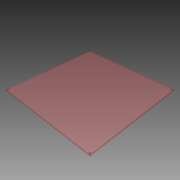
# Autodesk Inventor part: pcb_heatbed
Saved by Autodesk Inventor 2014 (Build 180170000, 170)
## iProperties
Created: 2013-11-29
Part Number: pcb_heatbed
Material: Generic
Document SubType Name: Modeling
Designer: buben
Density: 1 g/cm^3
Appearance: pcb_red
Author: buben
Autodesk Inventor part; units mm, degrees
ref_plane "YZ Plane" through (0, 0, 0) normal (1, 0, 0) x (0, 1, 0)
ref_plane "XZ Plane" through (0, 0, 0) normal (0, 1, 0) x (-1, 0, 0)
ref_plane "XY Plane" through (0, 0, 0) normal (0, 0, 1) x (1, 0, 0)
sketch "Sketch1" plane through (0, 0, 0) normal (0, 0, 1) x (1, 0, 0)
  line L0 (0, 0) -> (214, 0)
  line L1 (214, 0) -> (214, 214)
  line L2 (214, 214) -> (0, 214)
  line L3 (0, 214) -> (0, 0)
  line L4 (2.5, 211.5) -> (211.5, 211.5) construction
  line L5 (211.5, 211.5) -> (211.5, 2.5) construction
  line L6 (211.5, 2.5) -> (2.5, 2.5) construction
  line L7 (2.5, 2.5) -> (2.5, 211.5) construction
  circle A0 centre (2.5, 211.5) radius 1.7
  circle A1 centre (211.5, 211.5) radius 1.7
  circle A2 centre (211.5, 2.5) radius 1.7
  circle A3 centre (2.5, 2.5) radius 1.7
  point P0 (2.5, 107)
  point P1 (0, 107)
  point P2 (107, 211.5)
  point P3 (107, 214)
  dimension "d0" = 214
  dimension "d1" = 214
  dimension "d2" = 3.4
  dimension "d3" = 3.4
  dimension "d4" = 3.4
  dimension "d5" = 3.4
  dimension "d6" = 209
  dimension "d7" = 209
  constraints: 16 end point, 4 centre point, 4 coincident, 4 midpoint, 4 parallel, 2 horizontal, 2 perpendicular, 1 horizontal alignment, 1 vertical alignment
  measures "d0" distance of L0.start L0.end
  measures "d1" distance of L2.end L0.start
  measures "d2" diameter of A3
  measures "d3" diameter of A2
  measures "d4" diameter of A1
  measures "d5" diameter of A0
  measures "d6" distance of L4.start L4.end
  measures "d7" distance of L6.end L4.start
extrude "Extrusion1" add sketch "Sketch1" along normal blind 2
body "Solid1"
